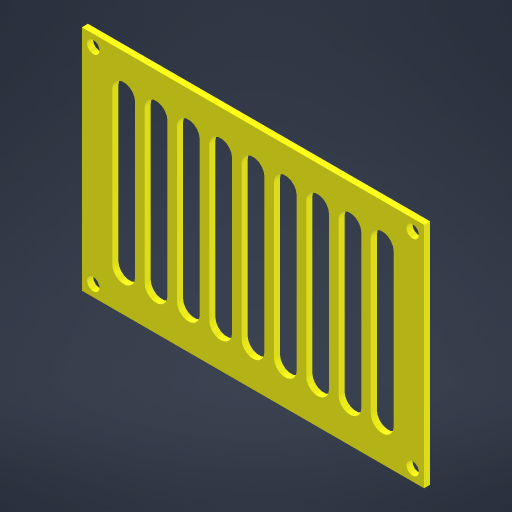
# Autodesk Inventor part: IntakeFilterBottom
Saved by Autodesk Inventor 2024.2 (Build 282272000, 272)
## iProperties
Created: 2024-06-05
Part Number: IntakeFilterBottom
Material: PBT Plastic
Document SubType Name: Modeling
Designer: simon
Density: 1.31 g/cm^3
Appearance: Yellow
Author: simon
Autodesk Inventor part; units mm, degrees
ref_plane "YZ Plane" through (0, 0, 0) normal (1, 0, 0) x (0, 1, 0)
ref_plane "XZ Plane" through (0, 0, 0) normal (0, 1, 0) x (-1, 0, 0)
ref_plane "XY Plane" through (0, 0, 0) normal (0, 0, 1) x (1, 0, 0)
sketch "Sketch1" plane through (0, 0, 0) normal (0, 0, 1) x (1, 0, 0)
  line L0 (0, 0) -> (90, 0)
  line L1 (90, 0) -> (90, 60)
  line L2 (90, 60) -> (0, 60)
  line L3 (0, 60) -> (0, 0)
  dimension "d0" = 90
  dimension "d1" = 60
  constraints: 8 end point, 2 parallel, 1 horizontal, 1 perpendicular
  measures "d0" distance of L2.end L1.end
  measures "d1" distance of L1.end L0.end
extrude "Extrusion1" add sketch "Sketch1" along normal blind 1.6
sketch "Sketch2" plane through (0, 0, 0) normal (0, 0, -1) x (-1, 0, 0)
  circle A0 centre (-3, 3) radius 1.65 projected
  circle A1 centre (-3, 3) radius 1.65 projected
  line L0 (-14, 50) -> (-14, 10) projected
  arc A2 (-14, 10) -> (-8, 10) centre (-11, 10) ccw projected
  line L1 (-48, 50) -> (-48, 10) projected
  arc A3 (-48, 10) -> (-42, 10) centre (-45, 10) ccw projected
  line L2 (-42, 10) -> (-42, 50) projected
  arc A4 (-42, 50) -> (-48, 50) centre (-45, 50) ccw projected
  line L3 (-39.5, 50) -> (-39.5, 10) projected
  arc A5 (-39.5, 10) -> (-33.5, 10) centre (-36.5, 10) ccw projected
  line L4 (-33.5, 10) -> (-33.5, 50) projected
  arc A6 (-33.5, 50) -> (-39.5, 50) centre (-36.5, 50) ccw projected
  line L5 (-31, 50) -> (-31, 10) projected
  arc A7 (-31, 10) -> (-25, 10) centre (-28, 10) ccw projected
  line L6 (-25, 10) -> (-25, 50) projected
  arc A8 (-25, 50) -> (-31, 50) centre (-28, 50) ccw projected
  line L7 (-22.5, 50) -> (-22.5, 10) projected
  arc A9 (-22.5, 10) -> (-16.5, 10) centre (-19.5, 10) ccw projected
  line L8 (-16.5, 10) -> (-16.5, 50) projected
  arc A10 (-16.5, 50) -> (-22.5, 50) centre (-19.5, 50) ccw projected
  line L9 (-8, 10) -> (-8, 50) projected
  arc A11 (-8, 50) -> (-14, 50) centre (-11, 50) ccw projected
  line L10 (-14, 50) -> (-14, 10) projected
  arc A12 (-14, 10) -> (-8, 10) centre (-11, 10) ccw projected
  line L11 (-65, 50) -> (-65, 10) projected
  arc A13 (-65, 10) -> (-59, 10) centre (-62, 10) ccw projected
  line L12 (-59, 10) -> (-59, 50) projected
  arc A14 (-59, 50) -> (-65, 50) centre (-62, 50) ccw projected
  line L13 (-73.5, 50) -> (-73.5, 10) projected
  arc A15 (-73.5, 10) -> (-67.5, 10) centre (-70.5, 10) ccw projected
  line L14 (-67.5, 10) -> (-67.5, 50) projected
  arc A16 (-67.5, 50) -> (-73.5, 50) centre (-70.5, 50) ccw projected
  line L15 (-82, 50) -> (-82, 10) projected
  arc A17 (-82, 10) -> (-76, 10) centre (-79, 10) ccw projected
  line L16 (-76, 10) -> (-76, 50) projected
  arc A18 (-76, 50) -> (-82, 50) centre (-79, 50) ccw projected
  line L17 (-50.5, 10) -> (-50.5, 50) projected
  arc A19 (-50.5, 50) -> (-56.5, 50) centre (-53.5, 50) ccw projected
  line L18 (-56.5, 50) -> (-56.5, 10) projected
  arc A20 (-56.5, 10) -> (-50.5, 10) centre (-53.5, 10) ccw projected
  line L19 (-6, 5) -> (-84, 5) projected
  line L20 (-84, 5) -> (-84, 55) projected
  line L21 (-84, 55) -> (-6, 55) projected
  line L22 (-6, 55) -> (-6, 5) projected
  line L23 (-90, 0) -> (-90, 60) projected
  line L24 (-90, 60) -> (0, 60) projected
  line L25 (0, 60) -> (0, 0) projected
  line L26 (0, 0) -> (-90, 0) projected
  line L27 (-6, 5) -> (-6, 55) projected
  line L28 (-6, 55) -> (-84, 55) projected
  line L29 (-84, 55) -> (-84, 5) projected
  line L30 (-84, 5) -> (-6, 5) projected
  circle A21 centre (-87, 3) radius 1.65 projected
  circle A22 centre (-87, 57) radius 1.65 projected
  circle A23 centre (-3, 57) radius 1.65 projected
  circle A24 centre (-3, 3) radius 1.65 projected
extrude "Extrusion2" cut sketch "Sketch2" against normal blind 1.6 contours A0 | A11 L9 A2 L0 | A4 L2 A3 L1 | A6 L4 A5 L3 | A8 L6 A7 L5 | A10 L8 A9 L7 | A14 L12 A13 L11 | A16 L14 A15 L13 | A18 L16 A17 L15 | A20 L18 A19 L17 | A21 | A22 | A23
body "Solid1"
